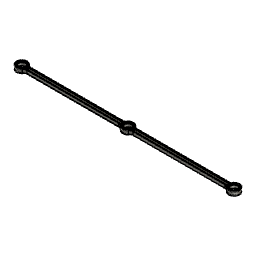
Main Wheel Link (Autodesk Fusion 360 design; units mm, degrees)
Autodesk Fusion 360 part; units mm, degrees
sketch "Sketch1" plane through (0, 0, 0) normal (0, 0, 1) x (1, 0, 0) in component "Component"
  circle A0 centre (0, 0) radius 1.55
  circle A1 centre (-50, 0) radius 1.55
  circle A2 centre (50, 0) radius 1.55
  circle A3 centre (0, 0) radius 2.25
  circle A4 centre (50, 0) radius 2.25
  circle A5 centre (-50, 0) radius 2.25
  line L0 (50, 0) -> (50, 1)
  line L1 (50, 0) -> (50, -1)
  circle A6 centre (0, 0) radius 2.5
  circle A7 centre (-50, 0) radius 2.5
  circle A8 centre (50, 0) radius 2.5
  circle A9 centre (50, 0) radius 1.75
  arc A10 (47.042, 0.5) -> (47.042, -0.5) centre (50, 0) ccw
  arc A11 (-2.958, 0.5) -> (-2.958, -0.5) centre (0, 0) ccw
  arc A12 (2.958, -0.5) -> (2.958, 0.5) centre (0, 0) ccw
  line L2 (47.042, -0.5) -> (2.958, -0.5)
  line L3 (2.958, 0.5) -> (47.042, 0.5)
  line L4 (47.7087, -1) -> (2.2913, -1)
  line L5 (2.2913, 1) -> (47.7087, 1)
  line L6 (-47.7087, 1) -> (-2.2913, 1)
  arc A13 (-47.042, -0.5) -> (-47.042, 0.5) centre (-50, 0) ccw
  line L7 (-2.958, -0.5) -> (-47.042, -0.5)
  line L8 (-47.042, 0.5) -> (-2.958, 0.5)
  line L9 (-2.2913, -1) -> (-47.7087, -1)
  circle A14 centre (0, 0) radius 1.75
  circle A15 centre (-50, 0) radius 1.75
  line L10 (-2.6458, -0.75) -> (-47.3542, -0.75)
  arc A16 (-47.3542, -0.75) -> (-47.3542, 0.75) centre (-50, 0) ccw
  line L11 (-47.3542, 0.75) -> (-2.6458, 0.75)
  arc A17 (-2.6458, 0.75) -> (-2.6458, -0.75) centre (0, 0) ccw
  line L12 (47.3542, -0.75) -> (2.6458, -0.75)
  arc A18 (2.6458, -0.75) -> (2.6458, 0.75) centre (0, 0) ccw
  line L13 (2.6458, 0.75) -> (47.3542, 0.75)
  arc A19 (47.3542, 0.75) -> (47.3542, -0.75) centre (50, 0) ccw
  dimension "d1" = 3.1
  dimension "d4" = 50
  dimension "d5" = 0
  dimension "d6" = 50
  dimension "d7" = 50
  dimension "d8" = 4.5
  dimension "d9" = 4.5
  dimension "d10" = 4.5
  dimension "d13" = 1
  dimension "d14" = 1
  dimension "d16" = 5
  dimension "d17" = 5
  dimension "d20" = 5
  dimension "d21" = 3.5
  dimension "d25" = 3.5
  dimension "d26" = 3.5
  dimension "d27" = -0.25
  dimension "d28" = -0.25
  constraint coincident A0.centre A3.centre
  constraint concentric A2 A4
  constraint concentric A1 A5
  constraint coincident A2.centre A4.centre
  constraint vertical L0
  constraint parallel L0 L1
  constraint concentric A3 A6
  constraint concentric A5 A7
  constraint concentric A2 A8
  constraint concentric A8 A9
  constraint concentric A8 A10
  constraint coincident A8 L5.end
  constraint coincident A8 L4.start
  constraint concentric A6 A11
  constraint concentric A11 A12
  constraint coincident A11.end L2
  constraint collinear L2 L7
  constraint collinear L4 L9
  constraint coincident A6 L9.start
  constraint coincident A6 L4.end
  constraint collinear L5 L6
  constraint coincident A6 L6.end
  constraint coincident A6 L5.start
  constraint concentric A7 A13
  constraint coincident A7 L6.start
  constraint coincident A7 L9.end
  constraint concentric A12 A14
  constraint concentric A1 A15
  measures "d1" diameter of A0
  measures "d6" distance of A0.centre A1.centre
  measures "d7" distance of A0.centre A2.centre
  measures "d8" diameter of A3
  measures "d9" diameter of A4
  measures "d10" diameter of A5
  measures "d13" distance of A2.centre L0.end
  measures "d14" distance of A2.centre L1.end
  measures "d16" diameter of A6
  measures "d17" diameter of A7
  measures "d20" diameter of A8
  measures "d21" diameter of A9
  measures "d25" diameter of A14
  measures "d26" diameter of A15
extrude "Extrude1" add sketch "Sketch1" along normal blind 2 contours A6 | A8 | A7 makes body 1 at (2.4876, 0.2489, 1.3333) makes body 2 at (52.4876, 0.2489, 1.3333) makes body 3 at (-47.5124, 0.2489, 1.3333) in component "Component"
extrude "Extrude2" add sketch "Sketch1" along normal blind 1.75 separate body contours A9 | A14 | A15 makes body 4 at (-51.158, -1.3121, 1.1667) makes body 5 at (1.7413, -0.1742, 1.1667) makes body 6 at (48.842, -1.3121, 1.1667) in component "Component"
extrude "Extrude3" cut sketch "Sketch1" along normal blind 0.25 contours A9 | A14 | A15 bodies 4 5 6 in component "Component"
extrude "Extrude4" add sketch "Sketch1" along normal blind 1.5 contours A3 | A4 | A5 bodies 1 2 3 4 5 6 in component "Component"
extrude "Extrude5" cut sketch "Sketch1" along normal blind 0.5 contours A3 | A4 | A5 bodies 1 2 3 in component "Component"
extrude "Extrude6" add sketch "Sketch1" along normal blind 1.75 contours A6 A8 L4 L5 | A6 A7 L6 L9 bodies 1 2 3 in component "Component"
extrude "Extrude7" cut sketch "Sketch1" along normal blind 0.25 contours A6 A8 L4 L5 | A6 A7 L6 L9 bodies 1 in component "Component"
extrude "Extrude8" add sketch "Sketch1" along normal blind 1.5 contours L10 A16 L11 A17 | L12 A18 L13 A19 bodies 1 in component "Component"
extrude "Extrude9" cut sketch "Sketch1" along normal blind 0.5 contours L10 A16 L11 A17 bodies 1 in component "Component"
extrude "Extrude10" add sketch "Sketch1" along normal blind 1.625 contours A10 A12 L2 L3 | A11 A13 L7 L8 bodies 1 in component "Component"
extrude "Extrude11" cut sketch "Sketch1" along normal blind 0.375 contours A10 A12 L2 L3 | A11 A13 L7 L8 bodies 1 in component "Component"
fillet "Fillet1" radius 2 8 edges at (2.2913, -1, 1) (-2.2913, -1, 1) (47.7087, -1, 1) (47.7087, 1, 1) (2.2913, 1, 1) (-47.7087, 1, 1) (-47.7087, -1, 1) (-2.2913, 1, 1) on bodies 1 in component "Component"
component "Component" placed x (1, 0, 0) y (0, 1, 0) z (0, 0, 1) at (0, 0, 0)
